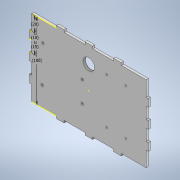
# Autodesk Inventor part: крепления
Saved by Autodesk Inventor 2021 (Build 250183000, 183)
## iProperties
Created: 2021-04-11
Part Number: крепления
Material: Типовые
Document SubType Name: Modeling
Designer: user
Density: 1 g/cm^3
Appearance: По умолчанию
Author: user
Autodesk Inventor part; units mm, degrees
ref_plane "YZ Plane" through (0, 0, 0) normal (1, 0, 0) x (0, 1, 0)
ref_plane "XZ Plane" through (0, 0, 0) normal (0, 1, 0) x (-1, 0, 0)
ref_plane "XY Plane" through (0, 0, 0) normal (0, 0, 1) x (1, 0, 0)
sketch "Эскиз1" plane through (0, 0, 0) normal (0, 0, 1) x (1, 0, 0)
  line L0 (0, 53) -> (5, 53)
  line L1 (5, 53) -> (5, 50)
  line L2 (32.5, 53) -> (42.5, 53)
  line L3 (42.5, 53) -> (42.5, 50)
  line L4 (32.5, 50) -> (32.5, 53)
  line L5 (78, 30) -> (75, 30)
  line L6 (75, 20) -> (78, 20)
  line L7 (78, 20) -> (78, 30)
  line L8 (78, 5) -> (75, 5)
  line L9 (78, 0) -> (78, 5)
  line L10 (5, 50) -> (32.5, 50)
  line L11 (42.5, 50) -> (75, 50)
  line L12 (5, 50) -> (32.5, 50)
  line L13 (42.5, 50) -> (75, 50)
  line L14 (75, 50) -> (75, 30)
  line L15 (75, 20) -> (75, 5)
  line L16 (75, 50) -> (75, 30)
  line L17 (75, 20) -> (75, 5)
  line L18 (0, -53) -> (5, -53)
  line L19 (5, -53) -> (5, -50)
  line L20 (32.5, -53) -> (42.5, -53)
  line L21 (42.5, -53) -> (42.5, -50)
  line L22 (32.5, -50) -> (32.5, -53)
  line L23 (78, -30) -> (75, -30)
  line L24 (75, -20) -> (78, -20)
  line L25 (78, -20) -> (78, -30)
  line L26 (78, -5) -> (75, -5)
  line L27 (78, 0) -> (78, -5)
  line L28 (5, -50) -> (32.5, -50)
  line L29 (42.5, -50) -> (75, -50)
  line L30 (5, -50) -> (32.5, -50)
  line L31 (42.5, -50) -> (75, -50)
  line L32 (75, -50) -> (75, -30)
  line L33 (75, -20) -> (75, -5)
  line L34 (75, -50) -> (75, -30)
  line L35 (75, -20) -> (75, -5)
  line L36 (0, 53) -> (-5, 53)
  line L37 (-5, 53) -> (-5, 50)
  line L38 (-32.5, 53) -> (-42.5, 53)
  line L39 (-42.5, 53) -> (-42.5, 50)
  line L40 (-32.5, 50) -> (-32.5, 53)
  line L41 (-78, 30) -> (-75, 30)
  line L42 (-75, 20) -> (-78, 20)
  line L43 (-78, 20) -> (-78, 30)
  line L44 (-78, 5) -> (-75, 5)
  line L45 (-78, 0) -> (-78, 5)
  line L46 (-5, 50) -> (-32.5, 50)
  line L47 (-42.5, 50) -> (-75, 50)
  line L48 (-5, 50) -> (-32.5, 50)
  line L49 (-42.5, 50) -> (-75, 50)
  line L50 (-75, 50) -> (-75, 30)
  line L51 (-75, 20) -> (-75, 5)
  line L52 (-75, 50) -> (-75, 30)
  line L53 (-75, 20) -> (-75, 5)
  line L54 (-32.5, -53) -> (-42.5, -53)
  line L55 (-32.5, -50) -> (-32.5, -53)
  line L56 (-5, -50) -> (-32.5, -50)
  line L57 (-5, -50) -> (-32.5, -50)
  line L58 (-5, -53) -> (-5, -50)
  line L59 (0, -53) -> (-5, -53)
  line L60 (-42.5, -53) -> (-42.5, -50)
  line L61 (-42.5, -50) -> (-75, -50)
  line L62 (-42.5, -50) -> (-75, -50)
  line L63 (-75, -50) -> (-75, -30)
  line L64 (-75, -50) -> (-75, -30)
  line L65 (-78, -30) -> (-75, -30)
  line L66 (-75, -20) -> (-78, -20)
  line L67 (-78, -20) -> (-78, -30)
  line L68 (-75, -20) -> (-75, -5)
  line L69 (-75, -20) -> (-75, -5)
  line L70 (-78, -5) -> (-75, -5)
  line L71 (-78, 0) -> (-78, -5)
  circle A0 centre (23.5, 30) radius 1
  circle A1 centre (48.5, 30) radius 1
  circle A2 centre (23.5, -30) radius 1
  circle A3 centre (48.5, -30) radius 1
  circle A4 centre (-60, 24) radius 1.5
  circle A5 centre (-61, -24) radius 1.5
  circle A6 centre (-8.5, -19) radius 1.5
  circle A7 centre (-8.5, 8.5) radius 1.5
  circle A8 centre (0, 30) radius 7.5
  point P0 (37.5, 50)
  point P1 (75, 25)
  point P2 (37.5, -50)
  point P3 (75, -25)
  point P4 (-37.5, 50)
  point P5 (-37.5, -50)
  point P6 (36, 0)
  dimension "d48" = 15
  constraints: 144 end point, 9 centre point, 6 horizontal, 6 perpendicular, 4 collinear, 2 parallel
  measures "d48" diameter of A8
extrude "Выдавливание3" add sketch "Эскиз1" along normal blind 3
sketch "Эскиз3" plane through (0, 0, 3) normal (0, 0, 1) x (1, 0, 0)
  line L0 (-75, 30) -> (-78, 30) projected
  line L1 (-42.5, 50) -> (-75, 50) projected
  line L2 (-78, 20) -> (-75, 20) projected
  line L3 (-75, 5) -> (-78, 5) projected
  line L4 (-75, -50) -> (-42.5, -50) projected
  point P0 (0, 0)
  dimension "d51" = 20
  dimension "d52" = 10
  dimension "d53" = 15
  dimension "d54" = 100
  measures "d51" distance between parallel lines of L0 L1
  measures "d52" distance between parallel lines of L2 L0
  measures "d53" distance between parallel lines of L3 L2
  measures "d54" distance between parallel lines of L4 L1
